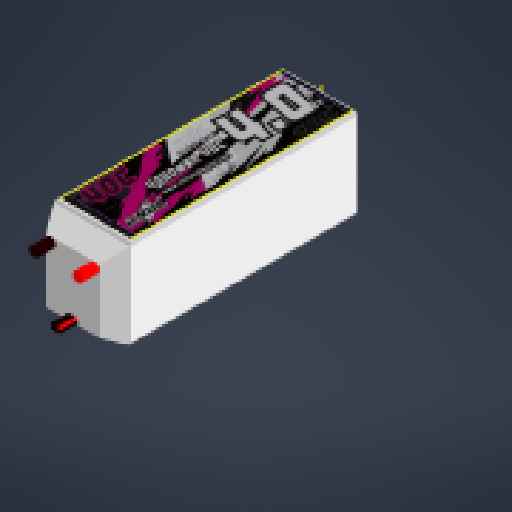
# Autodesk Inventor part: Lipo Battery CNHL 4000mAh
Saved by Autodesk Inventor 2026.1 (Build 301233000, 233)
## iProperties
Created: 2026-06-30
Part Number: Lipo Battery CNHL 4000mAh
Material: Generic
Document SubType Name: Modeling
Designer: adria
Density: 1 g/cm^3
Appearance: Default
Author: adria
Autodesk Inventor part; units mm, degrees
ref_plane "YZ Plane" through (0, 0, 0) normal (1, 0, 0) x (0, 1, 0)
ref_plane "XZ Plane" through (0, 0, 0) normal (0, 1, 0) x (-1, 0, 0)
ref_plane "XY Plane" through (0, 0, 0) normal (0, 0, 1) x (1, 0, 0)
sketch "Sketch1" plane through (0, 0, 0) normal (0, 0, 1) x (1, 0, 0)
  line L0 (-23, 27) -> (23, 27)
  line L1 (23, 27) -> (23, -27)
  line L2 (23, -27) -> (-23, -27)
  line L3 (-23, -27) -> (-23, 27)
  line L4 (-23, 27) -> (23, -27) construction
  line L5 (23, 27) -> (-23, -27) construction
  point P0 (0, 0)
  dimension "d0" = 46
  dimension "d1" = 54
  constraints: 12 end point, 2 midpoint, 2 parallel, 1 horizontal, 1 perpendicular
  measures "d0" distance of L1.end L2.end
  measures "d1" distance of L0.end L1.end
extrude "Extrusion1" add sketch "Sketch1" along normal blind 137
fillet "Fillet1" radius 2 9 edges at (-23, 27, 68.5) (0, 27, 137) (23, 27, 68.5) (0, 27, 0) (23, -27, 68.5) (23, 0, 0) (-23, 0, 0) (-23, -27, 68.5) (0, -27, 0)
sketch "Sketch2" plane through (-23, 27, 0) normal (0, 1, 0) x (1, 0, 0)
  line L0 (2, -131.2678) -> (2, -4.2112) construction
  line L1 (2, -4.2112) -> (44, -4.2112) construction
  line L2 (44, -4.2112) -> (44, -131.2678) construction
  line L3 (44, -131.2678) -> (2, -131.2678) construction
  line L4 (2, -135) -> (2, -2) projected
  line L5 (44, -2) -> (44, -135) projected
  point P0 (23, 0)
  constraints: 3 point on line, 2 other
sketch "Sketch3" plane through (0, 0, 137) normal (0, 0, 1) x (1, 0, 0)
  arc A0 (-23, -25) -> (-21, -27) centre (-21, -25) ccw projected
  line L0 (-21, -27) -> (21, -27) projected
  arc A1 (21, -27) -> (23, -25) centre (21, -25) ccw projected
  line L1 (23, -25) -> (23, 25) projected
  line L2 (-23, 25) -> (23, 25) projected
  line L3 (-23, 25) -> (-23, -25) projected
  point P0 (0, 0)
extrude "Extrusion2" add sketch "Sketch3" along normal blind 12 draft -30
sketch "Sketch4" plane through (0, 0, 149) normal (0, 0, 1) x (1, 0, 0)
  circle A0 centre (-13.0718, 15.0718) radius 3
  circle A1 centre (-13.0718, -17.0718) radius 3
  line L0 (-16.0718, 18.0718) -> (16.0718, 18.0718) projected
  line L1 (-16.0718, -20.0718) -> (-16.0718, 18.0718) projected
  line L2 (16.0718, 18.0718) -> (16.0718, -20.0718) projected
  circle A2 centre (13.0718, 0) radius 1
  circle A3 centre (15.0718, 0) radius 1
  circle A4 centre (15.0718, 2) radius 1
  circle A5 centre (13.0718, 2) radius 1
  line L3 (16.0718, -20.0718) -> (-16.0718, -20.0718) projected
  circle A6 centre (13.0718, -2) radius 1
  circle A7 centre (15.0718, -2) radius 1
  line L4 (0, 0) -> (13.0718, 0) construction
  point P0 (13.0718, 1)
  point P1 (14.0718, 2)
  point P2 (15.0718, 1)
  point P3 (14.0718, 0)
  point P4 (14.0718, -2)
  dimension "d45" = 6
  dimension "d46" = 6
  dimension "d48" = 2
  constraints: 14 tangent, 8 centre point, 5 equal radius, 2 end point, 1 horizontal, 1 horizontal alignment
  measures "d45" diameter of A0
  measures "d46" diameter of A1
  measures "d48" diameter of A3
extrude "Extrusion3" add sketch "Sketch4" along normal blind 10 contours A0 | A1 | A4 | A3 | A5 | A7 | A2 | A6
body "Solid1"
